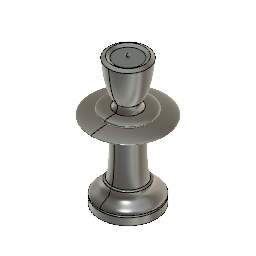
drottning skák verkefni 3 (v1~recovered) (Autodesk Fusion 360 design; units mm, degrees)
Autodesk Fusion 360 part; units mm, degrees
sketch "Sketch1" plane through (0, 0, 0) normal (1, 0, 0) x (0, 1, 0)
  line L0 (0, 0) -> (-8, 0)
  line L1 (-8, 0) -> (-8, 2)
  spline S0 degree 5 poles (-8, 2) (-8, 2.0073) (-7.9987, 2.0215) (-7.993, 2.0422) (-7.9776, 2.0683) (-7.946, 2.0983) (-7.9027, 2.1259) (-7.8503, 2.151) (-7.7926, 2.1739) (-7.7361, 2.1947) (-7.6882, 2.2141) (-7.6558, 2.2323) (-7.6443, 2.25) (-7.6558, 2.2677) (-7.6882, 2.2859) (-7.7361, 2.3053) (-7.7926, 2.3261) (-7.8503, 2.349) (-7.9027, 2.3741) (-7.946, 2.4017) (-7.9776, 2.4317) (-7.993, 2.4578) (-7.9987, 2.4785) (-8, 2.4927) (-8, 2.5) knots 0 0 0 0 0 0 0.05 0.1 0.15 0.2 0.25 0.3 0.35 0.4 0.45 0.5 0.55 0.6 0.65 0.7 0.75 0.8 0.85 0.9 0.95 1 1 1 1 1 1
  spline S1 degree 5 poles (-8, 2.5) (-7.9986, 2.5191) (-7.9934, 2.5579) (-7.9787, 2.6174) (-7.945, 2.6997) (-7.8788, 2.8075) (-7.7876, 2.9202) (-7.6697, 3.0378) (-7.523, 3.1603) (-7.3458, 3.2877) (-7.1377, 3.4204) (-6.9008, 3.5591) (-6.6409, 3.7051) (-6.3675, 3.8605) (-6.092, 4.0276) (-5.8269, 4.2086) (-5.5845, 4.406) (-5.3751, 4.6215) (-5.2061, 4.8565) (-5.0816, 5.1113) (-5.0036, 5.3861) (-4.9788, 5.6219) (-4.9813, 5.8075) (-4.9922, 5.9352) (-5, 6) knots 0 0 0 0 0 0 0.05 0.1 0.15 0.2 0.25 0.3 0.35 0.4 0.45 0.5 0.55 0.6 0.65 0.7 0.75 0.8 0.85 0.9 0.95 1 1 1 1 1 1
  spline S2 degree 5 poles (-5, 6) (-5.0009, 6.0102) (-5.0017, 6.0303) (-4.9999, 6.0593) (-4.9918, 6.0956) (-4.9711, 6.137) (-4.9391, 6.174) (-4.8949, 6.2062) (-4.8382, 6.2336) (-4.7697, 6.2565) (-4.6903, 6.275) (-4.6188, 6.2868) (-4.561, 6.294) (-4.5206, 6.2981) (-4.5, 6.3) knots 0 0 0 0 0 0 0.1 0.2 0.3 0.4 0.5 0.6 0.7 0.8 0.9 1 1 1 1 1 1
  spline S3 degree 5 poles (-4.5, 6.3) (-4.4647, 6.4266) (-4.3964, 6.6947) (-4.3012, 7.1416) (-4.1892, 7.8283) (-4.0751, 8.8466) (-3.9886, 10.0341) (-3.93, 11.3938) (-3.8978, 12.9155) (-3.8894, 14.5831) (-3.902, 16.3803) (-3.9273, 17.9111) (-3.9541, 19.1079) (-3.9754, 19.9269) (-3.987, 20.3418) knots 0 0 0 0 0 0 0.1 0.2 0.3 0.4 0.5 0.6 0.7 0.8 0.9 1 1 1 1 1 1
  spline S4 degree 5 poles (-3.987, 20.3418) (-4.439, 20.3897) (-5.3077, 20.4848) (-6.5042, 20.6252) (-7.8832, 20.8078) (-9.2208, 21.028) (-10.1346, 21.2394) (-10.5844, 21.441) (-10.5391, 21.6323) (-10.0039, 21.8133) (-9.01, 21.9847) (-7.875, 22.1147) (-6.8443, 22.2085) (-6.0786, 22.2693) (-5.6762, 22.2993) knots 0 0 0 0 0 0 0.1 0.2 0.3 0.4 0.5 0.6 0.7 0.8 0.9 1 1 1 1 1 1
  spline S5 degree 5 poles (-5.6762, 22.2993) (-5.7746, 22.3563) (-5.9582, 22.4676) (-6.1937, 22.626) (-6.4267, 22.8204) (-6.5748, 23.0333) (-6.5699, 23.2141) (-6.405, 23.3615) (-6.0845, 23.4762) (-5.6215, 23.5611) (-5.0301, 23.6191) (-4.4642, 23.646) (-3.9912, 23.656) (-3.6546, 23.6583) (-3.481, 23.6583) knots 0 0 0 0 0 0 0.1 0.2 0.3 0.4 0.5 0.6 0.7 0.8 0.9 1 1 1 1 1 1
  spline S6 degree 5 poles (-3.481, 23.6583) (-3.453, 23.6894) (-3.3987, 23.752) (-3.3221, 23.8475) (-3.2297, 23.978) (-3.1316, 24.1464) (-3.0525, 24.3209) (-2.9938, 24.5017) (-2.9564, 24.6892) (-2.9395, 24.8832) (-2.9414, 25.0831) (-2.9568, 25.2473) (-2.9756, 25.3728) (-2.9913, 25.4574) (-3, 25.5) knots 0 0 0 0 0 0 0.1 0.2 0.3 0.4 0.5 0.6 0.7 0.8 0.9 1 1 1 1 1 1
  spline S7 degree 5 poles (-3, 25.5) (-3.0809, 25.6251) (-3.2399, 25.8821) (-3.4699, 26.2884) (-3.7591, 26.8721) (-4.0899, 27.6762) (-4.3878, 28.5603) (-4.6509, 29.5286) (-4.8797, 30.58) (-5.0768, 31.7082) (-5.2452, 32.9058) (-5.3592, 33.9143) (-5.4338, 34.697) (-5.4787, 35.2304) (-5.5, 35.5) knots 0 0 0 0 0 0 0.1 0.2 0.3 0.4 0.5 0.6 0.7 0.8 0.9 1 1 1 1 1 1
  line L2 (0, 35.7) -> (0, 0)
  line L3 (0, 35.7) -> (0, 35.714)
  line L4 (-5.5, 35.5) -> (-4.5, 36)
  line L5 (-4.5, 36) -> (-3.6139, 35.5077)
  line L6 (-3.6139, 35.5077) -> (0, 35.5077)
  spline S8 degree 5 poles (-0.1902, 35.5077) (-0.1891, 35.5179) (-0.187, 35.538) (-0.1845, 35.5676) (-0.1824, 35.6058) (-0.1821, 35.6512) (-0.1844, 35.6941) (-0.1893, 35.7343) (-0.1971, 35.7717) (-0.2076, 35.8063) (-0.2207, 35.8384) (-0.233, 35.8622) (-0.2432, 35.8791) (-0.2505, 35.8899) (-0.2542, 35.8952) knots 0 0 0 0 0 0 0.1 0.2 0.3 0.4 0.5 0.6 0.7 0.8 0.9 1 1 1 1 1 1
  line L7 (0, 35.9125) -> (0, 35.5077)
  line L8 (0, 35.714) -> (0, 35.7)
  spline S9 degree 5 poles (-0.2542, 35.8952) (-0.2759, 35.9091) (-0.3171, 35.9367) (-0.3724, 35.9778) (-0.4331, 36.0319) (-0.4869, 36.0986) (-0.5183, 36.1639) (-0.5274, 36.2276) (-0.5155, 36.2891) (-0.4852, 36.3476) (-0.4403, 36.4022) (-0.3848, 36.4517) (-0.3229, 36.4953) (-0.258, 36.5323) (-0.1922, 36.5624) (-0.1269, 36.5856) (-0.0755, 36.5987) (-0.0375, 36.6055) (-0.0125, 36.6087) (0, 36.61) knots 0 0 0 0 0 0 0.066667 0.133333 0.2 0.266667 0.333333 0.4 0.466667 0.533333 0.6 0.666667 0.733333 0.8 0.866667 0.933333 1 1 1 1 1 1
  line L9 (0, 36.61) -> (0, 35.9125)
  line L10 (0, 0) -> (0, 17.754)
  point P0 (-7.85, 2.15)
  point P1 (-7.65, 2.25)
  point P2 (-7.85, 2.35)
  point P3 (-7.8, 2.9)
  point P4 (-7, 3.5)
  point P5 (-5.5, 4.5)
  point P6 (-4.9, 6.2)
  point P7 (-4, 10)
  point P8 (-10.5, 21.5)
  point P9 (-6.4973, 23.2536)
  point P10 (-3, 24.5)
  point P11 (-4.5, 29)
  point P12 (-0.1904, 35.7357)
  point P13 (-0.5217, 36.2364)
  point P14 (-0.318, 36.4963)
  dimension "d2" = 17.754
  dimension "d3" = 10.5
  constraint coincident L0.start L2.end
  constraint horizontal L0
  constraint perpendicular L0 L1
  constraint perpendicular L0 L2
  constraint coincident L2 L6.end
  constraint perpendicular L2 L6
  constraint coincident L6 S8.start
  constraint perpendicular L6 L7
  constraint parallel L2 L8
  constraint parallel L7 L9
  constraint perpendicular L0 L10
  measures "d2" distance of L0.start L10.end
  measures "d3" distance of P8 L2
revolve "Revolve1" add sketch "Sketch1" angle 360 about axis through (0, 0, 35.7) along (0, 0, -1) in component "Component'"
sketch "Sketch2" plane through (0, 0, 0) normal (1, 0, 0) x (0, 1, 0)
sketch "Sketch3" plane through (0, 0, 35.5077) normal (0, 0, 1) x (-1, 0, 0)
  circle A0 centre (0, 0) radius 3.6139
  circle A1 centre (0, 0) radius 0.1902
sketch "Sketch4" plane through (0, 0, 0) normal (1, 0, 0) x (0, 1, 0)
component "Component'" placed x (1, 0, 0) y (0, 1, 0) z (0, 0, 1) at (0, 0, 0)
